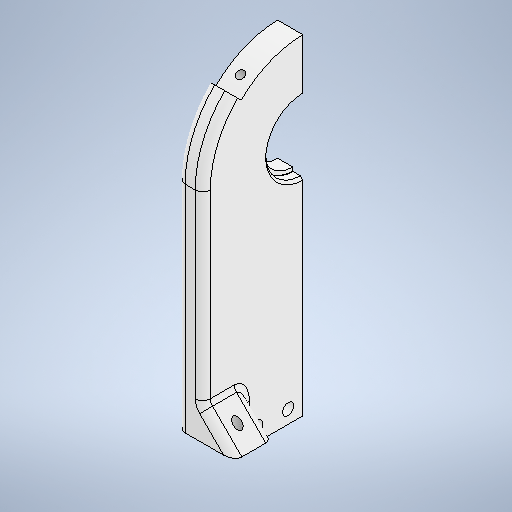
# Autodesk Inventor part: joint4_base_support_2
Saved by Autodesk Inventor 2025.3 (Build 293356030, 356C)
## iProperties
Created: 2025-11-08
Part Number: joint4_base_support_2
Material: PLA filament
Document SubType Name: Modeling
Designer: MSI
Density: 1.2 g/cm^3
Appearance: 일반
Mass: 52.6465 g
Surface Area: 138.203 cm^2
Volume: 43.8721 cm^3
Author: MSI
Autodesk Inventor part; units mm, degrees
ref_plane "YZ Plane" through (0, 0, 0) normal (1, 0, 0) x (0, 1, 0)
ref_plane "XZ Plane" through (0, 0, 0) normal (0, 1, 0) x (-1, 0, 0)
sketch "스케치1" plane through (0, 0, 0) normal (1, 0, 0) x (0, 1, 0)
  circle A0 centre (0, 0) radius 40
  line L0 (0, 40) -> (-96, 40)
  line L1 (-96, 40) -> (-96, -40)
  line L2 (-96, -40) -> (0, -40)
  line L3 (0, -40) -> (0, 40)
  point P0 (0, -40)
  point P1 (0, 40)
  dimension "d0" = 80
  dimension "d1" = 96
  dimension "d2" = 80
  constraints: 8 end point, 2 coincident, 2 parallel, 1 centre point, 1 horizontal, 1 midpoint, 1 perpendicular
  measures "d0" diameter of A0
  measures "d1" distance of L2.end L1.end
  measures "d2" distance of L1.end L0.end
extrude "돌출1" add sketch "스케치1" along normal mid plane 10
sketch "스케치2" plane through (5, 0, 0) normal (1, 0, 0) x (0, 0, -1)
  arc A0 (40, 0) -> (-40, 0) centre (0, 0) ccw projected
  constraints: 1 coincident
hole "구멍1" at (5, 0, 0) direction (-1, 0, 0) diameter 25 end through all counterbore diameter 28 counterbore depth 4
fillet "모깎기1" radius 0.1 1 edges at (1, 0, 14)
sketch "스케치3" plane through (-5, -96, 40) normal (0, 0, 1) x (1, 0, 0)
  line L0 (0, 0) -> (10, 0) projected
  line L1 (10, 0) -> (10, 96) projected
  line L2 (0, 0) -> (10, 0)
  line L3 (10, 0) -> (10, 10.5)
  line L4 (10, 10.5) -> (0, 10.5)
  line L5 (0, 10.5) -> (0, 0)
  point P0 (5, 96)
  dimension "d12" = 10.5
  constraints: 8 end point, 2 parallel, 1 horizontal, 1 perpendicular, 1 point on line
  measures "d12" distance between parallel lines of L0 L4
extrude "돌출2" cut sketch "스케치3" against normal blind 15.5
sketch "스케치5" plane through (-5, 0, 40) normal (0, 0, 1) x (1, 0, 0)
  line L0 (10, 0) -> (10, -85.5) projected
  line L1 (10, -73) -> (22.5, -85.5)
  line L2 (22.5, -85.5) -> (10, -85.5)
  point P0 (5, 0)
  dimension "d27" = 45
  dimension "d30" = 12.5
  constraints: 4 end point, 1 horizontal, 1 point on line
  measures "d27" angle of L2 L1
  measures "d30" distance from line of L2 L1.start
extrude "돌출3" add sketch "스케치5" against normal blind 15.5
mirror "미러1" about plane through (0, 0, 0) normal (0, 0, 1) of "돌출2", "돌출3"
sketch "스케치6" plane through (-5, -85.5, 24.5) normal (0, -1, 0) x (1, 0, 0)
  line L0 (5, 8) -> (16.25, 8)
  line L1 (16.25, 8) -> (16.25, -57)
  line L2 (16.25, -57) -> (5, -57)
  line L3 (5, -57) -> (5, 8)
  line L4 (0, 15.5) -> (10, 15.5) projected
  line L5 (22.5, 15.5) -> (10, 15.5) projected
  line L6 (22.5, -64.5) -> (10, -64.5) projected
  line L7 (10, -49) -> (10, -64.5) projected
  line L8 (10, -49) -> (22.5, -49) projected
  line L9 (22.5, -64.5) -> (22.5, -49) projected
  line L10 (22.5, 15.5) -> (10, 15.5) projected
  line L11 (22.5, 15.5) -> (22.5, 0) projected
  line L12 (10, 0) -> (22.5, 0) projected
  line L13 (10, 15.5) -> (10, 0) projected
  point P0 (5, -24.5)
  point P1 (5, 15.5)
  point P2 (16.25, 15.5)
  dimension "d44" = 7.5
  dimension "d45" = 7.5
  constraints: 8 end point, 4 coincident, 2 midpoint, 2 parallel, 2 point on line, 1 horizontal, 1 perpendicular
  measures "d44" distance between parallel lines of L0 L5
  measures "d45" distance between parallel lines of L2 L6
hole "구멍3" at (11.25, -85.5, -32.5) at (0, -85.5, -32.5) at (0, -85.5, 32.5) at (11.25, -85.5, 32.5) direction (0, 1, 0) diameter 3.242 depth 13 tip angle 118 thread size "M4x0.7" class "6H" standard "ISO Metric profile"
sketch "스케치4" plane through (-5, 0, 0) normal (-1, 0, 0) x (0, 0, 1)
  line L0 (-18.375, -90.75) -> (18.375, -90.75)
  line L1 (-24.5, -96) -> (24.5, -96) projected
  line L2 (-24.5, -85.5) -> (-24.5, -96) projected
  point P0 (0, 0)
  point P1 (0, -90.75)
  point P2 (0, -96)
  point P3 (-24.5, -90.75)
  point P4 (-6.125, -90.75)
  point P5 (6.125, -90.75)
  dimension "d17" = 36.75
  dimension "d18" = 12.25
  dimension "d19" = 12.25
  constraints: 3 midpoint, 3 point on line, 2 coincident, 2 end point, 1 horizontal, 1 vertical alignment
  measures "d17" distance of L0.start L0.end
  measures "d18" distance of point (-6.125, -90.75) point (-18.375, -90.75)
  measures "d19" distance of point (6.125, -90.75) point (18.375, -90.75)
hole "구멍2" at (-5, -90.75, -18.375) at (-5, -90.75, -6.125) at (-5, -90.75, 6.125) at (-5, -90.75, 18.375) direction (1, 0, 0) diameter 4.5 end through all counterbore diameter 8 counterbore depth 4.4 clearance for "Socket Head Cap Screw ISO 4762" size "M4" standard "ISO"
fillet "모깎기4" radius 3 2 edges at (11.25, -79.25, 24.5) (11.25, -79.25, -24.5)
fillet "모깎기2" radius 3 4 edges at (0, 0, 40) (0, 0, -40) (5, -73, 33.75) (5, -73, -33.75)
fillet "모깎기3" radius 3 6 edges at (-5, -42.75, -40) (-5, -42.75, 40) (-5, 40, 0) (5, -35.8787, 40) (5, -35.8787, -40) (5, 40, 0)
chamfer "모따기1" distance 1 angle 45 3 edges at (0, -96, 24.5) (0, -96, -24.5) (5, 0, 14)
sketch "스케치9" plane through (0, 0, 0) normal (1, 0, 0) x (0, 1, 0)
  arc A0 (0, -40) -> (0, 40) centre (0, 0) ccw
  line L0 (28.284271, 28.284271) -> (0, 0)
  line L1 (0, 0) -> (28.284271, -28.284271)
  line L2 (0, 0) -> (40, 0)
  arc A1 (0, -35) -> (0, 35) centre (0, 0) ccw
  point P0 (24.748737, -24.748737)
  point P1 (24.748737, 24.748737)
  dimension "d60" = 45
  dimension "d61" = 45
  dimension "d62" = 5
  constraints: 6 end point, 5 point on circle, 1 centre point
  measures "d60" angle of L2 L0
  measures "d61" angle of L1 L2
  measures "d62" radial gap between concentric circles of A0 A1
extrude "돌출5" cut sketch "스케치9" along normal mid plane 10 contours L1 A1 L2 A0 | L2 A1 L0 A0
sketch "스케치10" plane through (0, 0, 0) normal (1, 0, 0) x (0, 1, 0)
  line L0 (28.644537, 20.05712) -> (0, 0)
  arc A0 (24.748737, -24.748737) -> (24.748737, 24.748737) centre (0, 0) ccw
  line L1 (0, 0) -> (35, 0) construction
  dimension "d65" = 35
  constraints: 4 end point, 1 horizontal, 1 point on circle
  measures "d65" angle of L1 L0
ref_plane "작업 평면1" through (0, 28.644537, 20.05712) normal (0, -0.819152, -0.5735764) x (1, 0, 0)
sketch "스케치11" plane through (0, 28.644537, 20.05712) normal (0, -0.819152, -0.5735764) x (1, 0, 0)
  point P0 (0, 0)
  point P1 (0, 0)
  constraints: 1 coincident
hole "구멍5" at (0, 28.644537, 20.05712) direction (0, -0.819152, -0.5735764) diameter 3.242 depth 16 tip angle 118 thread size "M4x0.7" class "6H" standard "ISO Metric profile"
sketch "스케치12" plane through (0.652069, 29.495761, 18.841446) normal (0, -0.819152, -0.5735764) x (-1, 0, 0)
  circle A0 centre (0.652069, -1.484064) radius 1.621
  point P0 (0.652069, -1.484064)
  constraints: 1 centre point, 1 coincident
extrude "돌출6" cut sketch "스케치12" against normal through all
pattern_circular "원형 패턴1" count 2 over 70 about axis through (-153.101233, 0, 0) along (-1, 0, 0) of "구멍5", "돌출6"
sketch "스케치7" plane through (0, 0, 0) normal (1, 0, 0) x (0, 1, 0)
  line L0 (61.763617, 0.25) -> (-145.867981, 0.25)
  line L1 (-145.867981, 0.25) -> (-145.867981, 122.560008)
  line L2 (-145.867981, 122.560008) -> (61.763617, 122.560008)
  line L3 (61.763617, 122.560008) -> (61.763617, 0.25)
  point P0 (0, 0)
  dimension "d79" = 0.25
  constraints: 8 end point, 2 parallel, 1 horizontal, 1 perpendicular
  measures "d79" distance from line of point (0, 0) L0
extrude "돌출4" cut sketch "스케치7" along normal through all both and the other way through all keep common part
sketch "스케치8" plane through (-5, -96, 0.25) normal (0, 0, -1) x (-1, 0, 0)
  line L0 (-5, 121) -> (-5, 21)
  point P0 (-5, 96)
  point P1 (-5, 46)
  point P2 (-5, 71)
  dimension "d49" = 25
  dimension "d50" = 25
  dimension "d51" = 100
  dimension "d52" = 25
  constraints: 2 coincident, 2 end point, 2 point on line, 1 midpoint, 1 vertical
  measures "d49" distance of point (-5, 121) point (-5, 96)
  measures "d50" distance of point (-5, 71) point (-5, 96)
  measures "d51" distance of L0.start L0.end
  measures "d52" distance of point (-5, 71) point (-5, 46)
hole "구멍4" at (0, 25, 0.25) at (0, -75, 0.25) at (0, -50, 0.25) at (0, -25, 0.25) direction (0, 0, 1) diameter 5 depth 10 tip angle 118
equation "\"d45\" = d44"
equation "\"d17\" = 3 * d18"
equation "\"d19\" = d18"
equation "\"d61\" = d60"
equation "\"d50\" = d49"
equation "\"d51\" = 4 * d49"
equation "\"d52\" = d50"
